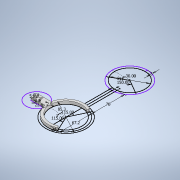
# Autodesk Inventor part: door mount backplate
Saved by Autodesk Inventor 2022 (Build 260153000, 153)
## iProperties
Created: 2021-11-11
Part Number: door mount backplate
Material: Generic
Document SubType Name: Modeling
Designer: a-dubs
Density: 1 g/cm^3
Appearance: Default
Author: a-dubs
Autodesk Inventor part; units mm, degrees
ref_plane "YZ Plane" through (0, 0, 0) normal (1, 0, 0) x (0, 1, 0)
ref_plane "XZ Plane" through (0, 0, 0) normal (0, 1, 0) x (-1, 0, 0)
ref_plane "XY Plane" through (0, 0, 0) normal (0, 0, 1) x (1, 0, 0)
sketch "Sketch1" plane through (0, 0, 0) normal (0, 1, 0) x (-1, 0, 0)
  circle A0 centre (0, 0) radius 32.5
  line L0 (0, 32.5) -> (0, 102.5)
  line L1 (0, 102.5) -> (0, 169.7)
  circle A1 centre (0, 136.1) radius 33.6
  circle A2 centre (0, 136.1) radius 42.65
  line L2 (42.65, 136.1) -> (40.15, 136.1)
  line L3 (40.15, 136.1) -> (62.55, 136.1)
  circle A3 centre (62.55, 136.1) radius 22.4
  line L4 (62.55, 136.1) -> (62.55, 134.2)
  line L5 (62.55, 136.1) -> (62.55, 138)
  circle A4 centre (62.55, 136.1) radius 2.8
  line L6 (62.55, 138) -> (64.6067, 138)
  line L7 (62.55, 138) -> (60.4933, 138)
  line L8 (62.55, 134.2) -> (60.4933, 134.2)
  line L9 (62.55, 134.2) -> (64.6067, 134.2)
  circle A5 centre (62.55, 136.1) radius 4.7
  line L10 (0, -32.5) -> (0, -37.5)
  circle A6 centre (0, 0) radius 37.5
  line L11 (0, 32.5) -> (5, 32.5)
  line L12 (5, 32.5) -> (5, 93.7441)
  line L13 (0, 32.5) -> (-5, 32.5)
  line L14 (-5, 32.5) -> (-5, 93.7441)
  line L15 (0, 0) -> (29.257, 0) construction
  line L16 (0, 0) -> (37.5, 0) construction
  line L17 (0, 0) -> (32.476, 18.75)
  line L18 (0, 0) -> (37.5, 0) construction
  line L19 (0, 0) -> (-32.476, 18.75)
  line L20 (0, 0) -> (37.5, 0) construction
  line L21 (0, 169.7) -> (0, 174.7)
  circle A7 centre (0, 136.1) radius 38.6
  line L22 (67.25, 136.1) -> (69.25, 136.1)
  line L23 (62.55, 140.8) -> (62.55, 142.8)
  line L24 (62.55, 131.4) -> (62.55, 129.4)
  line L25 (5, 93.7441) -> (5, 102.8741)
  line L26 (-5, 93.7441) -> (-5, 102.8741)
  line L27 (62.55, 129.4) -> (32.9252, 129.4)
  line L28 (62.55, 142.8) -> (32.9252, 142.8)
  line L29 (62.55, 142.8) -> (69.25, 142.8)
  line L30 (69.25, 142.8) -> (69.25, 136.1)
  line L31 (69.25, 129.4) -> (69.25, 136.1)
  line L32 (69.25, 129.4) -> (62.55, 129.4)
  line L33 (0, 136.1) -> (-18.0247, 97.446)
  line L34 (0, 136.1) -> (42.65, 136.1) construction
  line L35 (0, 136.1) -> (-18.0247, 174.754)
  line L36 (0, 136.1) -> (42.65, 136.1) construction
  point P0 (37.3613, 126.4)
  point P1 (41.8047, 144.5494)
  point P2 (41.8047, 127.6506)
  point P3 (42.1205, 129.4)
  point P4 (42.1205, 142.8)
  point P5 (5, 97.8252)
  point P6 (38.0141, 129.4)
  point P7 (41.1755, 129.4)
  point P8 (41.1755, 142.8)
  point P9 (38.0141, 142.8)
  point P10 (-5, 97.8252)
  point P11 (-16.3131, 171.0835)
  point P12 (-14.2, 166.5519)
  point P13 (-14.2, 105.6481)
  point P14 (-16.3131, 101.1165)
  dimension "d0" = 65
  dimension "d1" = 70
  dimension "d2" = 67.2
  dimension "d3" = 85.3
  dimension "d4" = 2.5
  dimension "d6" = 22.4
  dimension "d7" = 1.9
  dimension "d8" = 1.9
  dimension "d9" = 5.6
  dimension "d10" = 9.4
  dimension "d11" = 5
  dimension "d12" = 5
  dimension "d13" = 5
  dimension "d16" = 30
  dimension "d17" = 150
  dimension "d18" = 5
  dimension "d19" = 2
  dimension "d20" = 2
  dimension "d21" = 2
  dimension "d28" = 115
  dimension "d29" = 115
  constraints: 74 end point, 23 point on circle, 11 horizontal, 9 vertical, 8 equal length, 8 point on line, 7 centre point, 7 coincident, 4 perpendicular, 1 midpoint, 1 tangent, 3 other
  measures "d0" diameter of A0
  measures "d1" distance of L0.start L0.end
  measures "d2" distance of L0.end L1.end
  measures "d3" diameter of A2
  measures "d4" distance of L2.start L2.end
  measures "d6" distance of L2.end L3.end
  measures "d7" distance of L4.start L4.end
  measures "d8" distance of L4.start L5.end
  measures "d9" diameter of A4
  measures "d10" diameter of A5
  measures "d11" distance of L10.start L10.end
  measures "d12" distance of L0.start L11.end
  measures "d13" distance of L0.start L13.end
  measures "d16" angle of L18 L17
  measures "d17" angle of L20 L19
  measures "d18" distance of L1.end L21.end
  measures "d19" distance of L22.start L22.end
  measures "d20" distance of L23.start L23.end
  measures "d21" distance of L24.start L24.end
  measures "d28" angle of L33 L34
  measures "d29" angle of L36 L35
extrude "Extrusion1" add sketch "Sketch1" along normal blind 6 contours A7 L26 A1 L0 | L0 A1 L25 A7 | A7 L33 A1 L26 | L25 A1 L27 A7 | L27 A3 L2 A2 | A2 L3 A5 L24 L27 | L27 A7 L28 A3 | L27 A1 L28 A7 | A7 L21 A1 L35 | L2 A3 L28 A2 | A2 L28 L23 A5 L3 | L24 A5 L22 L31 L32 | L21 A7 L28 A1 | A5 | L29 L30 L22 A5 L23
chamfer "Chamfer1" distance 2 angle 45 1 edges at (-59.75, 0, 136.1)
fillet "Fillet1" radius 2 4 edges at (-69.25, 3, 129.4) (-69.25, 3, 142.8) (16.3131, 3, 101.1165) (16.3131, 3, 171.0835)
body "Solid1"
